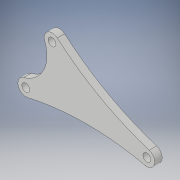
# Autodesk Inventor part: Part16
Saved by Autodesk Inventor 2019.2 (Build 232265000, 265)
## iProperties
Created: 2019-04-01
Part Number: Part16
Material: Generic
Document SubType Name: Modeling
Designer: richard.girt
Mass: 1.65683 g
Surface Area: 16.3203 cm^2
Volume: 1.65683 cm^3
Density: 1 g/cm^3
Appearance: Default
Author: richard.girt
Autodesk Inventor part; units mm, degrees
ref_plane "YZ Plane" through (0, 0, 0) normal (1, 0, 0) x (0, 1, 0)
ref_plane "XZ Plane" through (0, 0, 0) normal (0, 1, 0) x (-1, 0, 0)
ref_plane "XY Plane" through (0, 0, 0) normal (0, 0, 1) x (1, 0, 0)
sketch "Sketch1" plane through (0, 0, 0) normal (0, 0, 1) x (1, 0, 0)
  circle A0 centre (0, 0) radius 1.5
  circle A1 centre (10, 20) radius 1.5
  circle A2 centre (46, 0) radius 1.5
  arc A3 (11.9518, 22.2783) -> (7.2111, 18.8944) centre (10, 20) ccw
  arc A4 (-0.7889, 2.8944) -> (0.6699, -2.9242) centre (0, 0) ccw
  arc A5 (45.3301, -2.9242) -> (46.9032, 2.8608) centre (46, 0) ccw
  line L0 (11.4569, 22.6225) -> (47.4569, 2.6225) construction
  line L1 (46, -3) -> (0, -3) construction
  line L2 (-2.6833, 1.3416) -> (7.3167, 21.3416) construction
  line L3 (77.0115, 98.2206) -> (29.4569, 12.6225) construction
  line L4 (23, -100.3992) -> (23, -3) construction
  line L5 (-3.9443, 14.4721) -> (2.3167, 11.3416) construction
  arc A6 (11.9518, 22.2783) -> (46.9032, 2.8608) centre (77.0115, 98.2206) ccw
  arc A7 (-0.7889, 2.8944) -> (7.2111, 18.8944) centre (-3.9443, 14.4721) ccw
  arc A8 (45.3301, -2.9242) -> (0.6699, -2.9242) centre (23, -100.3992) ccw
  dimension "d0" = 3
  dimension "d1" = 10
  dimension "d2" = 20
  dimension "d3" = 46
  dimension "d4" = 0
  dimension "d5" = 6
  dimension "d6" = 12
  dimension "d7" = 100
  dimension "d8" = 100
  constraints: 18 point on circle, 12 end point, 9 centre point, 9 tangent, 7 coincident, 4 equal radius, 3 midpoint, 3 perpendicular
  measures "d0" diameter of A0
  measures "d1" horizontal distance of A1.centre point (0, 0)
  measures "d2" vertical distance of A1.centre point (0, 0)
  measures "d3" distance of A2.centre point (0, 0)
  measures "d4" vertical distance of point (0, 0) A2.centre
  measures "d5" diameter of A5
  measures "d6" radius of A7
  measures "d7" radius of A8
  measures "d8" radius of A6
extrude "Extrusion1" add sketch "Sketch1" along normal mid plane 2.8
body "Solid1"
